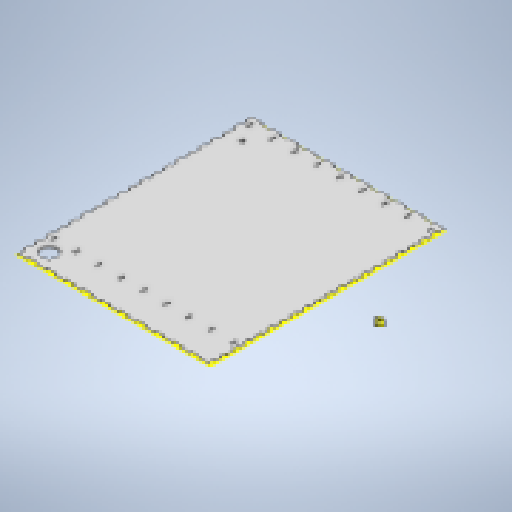
# Autodesk Inventor part: LedBoard
Saved by Autodesk Inventor 2024 (Build 280153000, 153)
## iProperties
Created: 2023-07-20
Part Number: LedBoard
Material: Generic
Document SubType Name: Modeling
Designer: Bruno
Density: 1 g/cm^3
Appearance: Default
Author: Bruno
Autodesk Inventor part; units mm, degrees
ref_plane "YZ Plane" through (0, 0, 0) normal (1, 0, 0) x (0, 1, 0)
ref_plane "XZ Plane" through (0, 0, 0) normal (0, 1, 0) x (-1, 0, 0)
ref_plane "XY Plane" through (0, 0, 0) normal (0, 0, 1) x (1, 0, 0)
sketch "Sketch1" plane through (0, 0, 0) normal (0, 1, 0) x (-1, 0, 0)
  line L0 (378.2704, -187.5) -> (378.2704, 177.5) projected
  line L1 (78.2704, -187.5) -> (378.2704, -187.5) projected
  line L2 (78.2704, 177.5) -> (78.2704, -187.5) projected
  line L3 (378.2704, 177.5) -> (78.2704, 177.5) projected
  line L4 (378.2704, 168.375) -> (378.2704, 177.5) projected
  line L5 (378.2704, 177.5) -> (375.2704, 177.5) projected
  line L6 (375.2704, 168.375) -> (375.2704, 177.5) projected
  line L7 (378.2704, 168.375) -> (375.2704, 168.375) projected
  line L8 (378.2704, 150.125) -> (378.2704, 159.25) projected
  line L9 (378.2704, 159.25) -> (375.2704, 159.25) projected
  line L10 (375.2704, 150.125) -> (375.2704, 159.25) projected
  line L11 (378.2704, 150.125) -> (375.2704, 150.125) projected
  line L12 (378.2704, 131.875) -> (378.2704, 141) projected
  line L13 (378.2704, 141) -> (375.2704, 141) projected
  line L14 (375.2704, 131.875) -> (375.2704, 141) projected
  line L15 (378.2704, 131.875) -> (375.2704, 131.875) projected
  line L16 (378.2704, 113.625) -> (378.2704, 122.75) projected
  line L17 (378.2704, 122.75) -> (375.2704, 122.75) projected
  line L18 (375.2704, 113.625) -> (375.2704, 122.75) projected
  line L19 (378.2704, 113.625) -> (375.2704, 113.625) projected
  line L20 (378.2704, 95.375) -> (378.2704, 104.5) projected
  line L21 (378.2704, 104.5) -> (375.2704, 104.5) projected
  line L22 (375.2704, 95.375) -> (375.2704, 104.5) projected
  line L23 (378.2704, 95.375) -> (375.2704, 95.375) projected
  line L24 (378.2704, 77.125) -> (378.2704, 86.25) projected
  line L25 (378.2704, 86.25) -> (375.2704, 86.25) projected
  line L26 (375.2704, 77.125) -> (375.2704, 86.25) projected
  line L27 (378.2704, 77.125) -> (375.2704, 77.125) projected
  line L28 (378.2704, 58.875) -> (378.2704, 68) projected
  line L29 (378.2704, 68) -> (375.2704, 68) projected
  line L30 (375.2704, 58.875) -> (375.2704, 68) projected
  line L31 (378.2704, 58.875) -> (375.2704, 58.875) projected
  line L32 (378.2704, 4.125) -> (378.2704, 13.25) projected
  line L33 (378.2704, 13.25) -> (375.2704, 13.25) projected
  line L34 (375.2704, 4.125) -> (375.2704, 13.25) projected
  line L35 (378.2704, 4.125) -> (375.2704, 4.125) projected
  line L36 (378.2704, 22.375) -> (378.2704, 31.5) projected
  line L37 (378.2704, 31.5) -> (375.2704, 31.5) projected
  line L38 (375.2704, 22.375) -> (375.2704, 31.5) projected
  line L39 (378.2704, 22.375) -> (375.2704, 22.375) projected
  line L40 (378.2704, 40.625) -> (378.2704, 49.75) projected
  line L41 (378.2704, 49.75) -> (375.2704, 49.75) projected
  line L42 (375.2704, 40.625) -> (375.2704, 49.75) projected
  line L43 (378.2704, 40.625) -> (375.2704, 40.625) projected
  line L44 (378.2704, -87.125) -> (378.2704, -78) projected
  line L45 (378.2704, -78) -> (375.2704, -78) projected
  line L46 (375.2704, -87.125) -> (375.2704, -78) projected
  line L47 (378.2704, -87.125) -> (375.2704, -87.125) projected
  line L48 (378.2704, -68.875) -> (378.2704, -59.75) projected
  line L49 (378.2704, -59.75) -> (375.2704, -59.75) projected
  line L50 (375.2704, -68.875) -> (375.2704, -59.75) projected
  line L51 (378.2704, -68.875) -> (375.2704, -68.875) projected
  line L52 (378.2704, -50.625) -> (378.2704, -41.5) projected
  line L53 (378.2704, -41.5) -> (375.2704, -41.5) projected
  line L54 (375.2704, -50.625) -> (375.2704, -41.5) projected
  line L55 (378.2704, -50.625) -> (375.2704, -50.625) projected
  line L56 (378.2704, -32.375) -> (378.2704, -23.25) projected
  line L57 (378.2704, -23.25) -> (375.2704, -23.25) projected
  line L58 (375.2704, -32.375) -> (375.2704, -23.25) projected
  line L59 (378.2704, -32.375) -> (375.2704, -32.375) projected
  line L60 (378.2704, -14.125) -> (378.2704, -5) projected
  line L61 (378.2704, -5) -> (375.2704, -5) projected
  line L62 (375.2704, -14.125) -> (375.2704, -5) projected
  line L63 (378.2704, -14.125) -> (375.2704, -14.125) projected
  line L64 (378.2704, -178.375) -> (378.2704, -169.25) projected
  line L65 (378.2704, -169.25) -> (375.2704, -169.25) projected
  line L66 (375.2704, -178.375) -> (375.2704, -169.25) projected
  line L67 (378.2704, -178.375) -> (375.2704, -178.375) projected
  line L68 (378.2704, -160.125) -> (378.2704, -151) projected
  line L69 (378.2704, -151) -> (375.2704, -151) projected
  line L70 (375.2704, -160.125) -> (375.2704, -151) projected
  line L71 (378.2704, -160.125) -> (375.2704, -160.125) projected
  line L72 (378.2704, -141.875) -> (378.2704, -132.75) projected
  line L73 (378.2704, -132.75) -> (375.2704, -132.75) projected
  line L74 (375.2704, -141.875) -> (375.2704, -132.75) projected
  line L75 (378.2704, -141.875) -> (375.2704, -141.875) projected
  line L76 (378.2704, -123.625) -> (378.2704, -114.5) projected
  line L77 (378.2704, -114.5) -> (375.2704, -114.5) projected
  line L78 (375.2704, -123.625) -> (375.2704, -114.5) projected
  line L79 (378.2704, -123.625) -> (375.2704, -123.625) projected
  line L80 (378.2704, -105.375) -> (378.2704, -96.25) projected
  line L81 (378.2704, -96.25) -> (375.2704, -96.25) projected
  line L82 (375.2704, -105.375) -> (375.2704, -96.25) projected
  line L83 (378.2704, -105.375) -> (375.2704, -105.375) projected
  line L84 (361.2704, -184.5) -> (347.2704, -184.5) projected
  line L85 (347.2704, -184.5) -> (347.2704, -187.5) projected
  line L86 (361.2704, -187.5) -> (347.2704, -187.5) projected
  line L87 (361.2704, -184.5) -> (361.2704, -187.5) projected
  line L88 (333.2704, -184.5) -> (319.2704, -184.5) projected
  line L89 (319.2704, -184.5) -> (319.2704, -187.5) projected
  line L90 (333.2704, -187.5) -> (319.2704, -187.5) projected
  line L91 (333.2704, -184.5) -> (333.2704, -187.5) projected
  line L92 (305.2704, -184.5) -> (291.2704, -184.5) projected
  line L93 (291.2704, -184.5) -> (291.2704, -187.5) projected
  line L94 (305.2704, -187.5) -> (291.2704, -187.5) projected
  line L95 (305.2704, -184.5) -> (305.2704, -187.5) projected
  line L96 (277.2704, -184.5) -> (263.2704, -184.5) projected
  line L97 (263.2704, -184.5) -> (263.2704, -187.5) projected
  line L98 (277.2704, -187.5) -> (263.2704, -187.5) projected
  line L99 (277.2704, -184.5) -> (277.2704, -187.5) projected
  line L100 (249.2704, -184.5) -> (235.2704, -184.5) projected
  line L101 (235.2704, -184.5) -> (235.2704, -187.5) projected
  line L102 (249.2704, -187.5) -> (235.2704, -187.5) projected
  line L103 (249.2704, -184.5) -> (249.2704, -187.5) projected
  line L104 (221.2704, -184.5) -> (207.2704, -184.5) projected
  line L105 (207.2704, -184.5) -> (207.2704, -187.5) projected
  line L106 (221.2704, -187.5) -> (207.2704, -187.5) projected
  line L107 (221.2704, -184.5) -> (221.2704, -187.5) projected
  line L108 (193.2704, -184.5) -> (179.2704, -184.5) projected
  line L109 (179.2704, -184.5) -> (179.2704, -187.5) projected
  line L110 (193.2704, -187.5) -> (179.2704, -187.5) projected
  line L111 (193.2704, -184.5) -> (193.2704, -187.5) projected
  line L112 (165.2704, -184.5) -> (151.2704, -184.5) projected
  line L113 (151.2704, -184.5) -> (151.2704, -187.5) projected
  line L114 (165.2704, -187.5) -> (151.2704, -187.5) projected
  line L115 (165.2704, -184.5) -> (165.2704, -187.5) projected
  line L116 (137.2704, -184.5) -> (123.2704, -184.5) projected
  line L117 (123.2704, -184.5) -> (123.2704, -187.5) projected
  line L118 (137.2704, -187.5) -> (123.2704, -187.5) projected
  line L119 (137.2704, -184.5) -> (137.2704, -187.5) projected
  line L120 (109.2704, -184.5) -> (95.2704, -184.5) projected
  line L121 (95.2704, -184.5) -> (95.2704, -187.5) projected
  line L122 (109.2704, -187.5) -> (95.2704, -187.5) projected
  line L123 (109.2704, -184.5) -> (109.2704, -187.5) projected
  line L124 (81.2704, -178.375) -> (81.2704, -169.25) projected
  line L125 (81.2704, -169.25) -> (78.2704, -169.25) projected
  line L126 (78.2704, -178.375) -> (78.2704, -169.25) projected
  line L127 (81.2704, -178.375) -> (78.2704, -178.375) projected
  line L128 (81.2704, -160.125) -> (81.2704, -151) projected
  line L129 (81.2704, -151) -> (78.2704, -151) projected
  line L130 (78.2704, -160.125) -> (78.2704, -151) projected
  line L131 (81.2704, -160.125) -> (78.2704, -160.125) projected
  line L132 (81.2704, -141.875) -> (81.2704, -132.75) projected
  line L133 (81.2704, -132.75) -> (78.2704, -132.75) projected
  line L134 (78.2704, -141.875) -> (78.2704, -132.75) projected
  line L135 (81.2704, -141.875) -> (78.2704, -141.875) projected
  line L136 (81.2704, -123.625) -> (81.2704, -114.5) projected
  line L137 (81.2704, -114.5) -> (78.2704, -114.5) projected
  line L138 (78.2704, -123.625) -> (78.2704, -114.5) projected
  line L139 (81.2704, -123.625) -> (78.2704, -123.625) projected
  line L140 (81.2704, -105.375) -> (81.2704, -96.25) projected
  line L141 (81.2704, -96.25) -> (78.2704, -96.25) projected
  line L142 (78.2704, -105.375) -> (78.2704, -96.25) projected
  line L143 (81.2704, -105.375) -> (78.2704, -105.375) projected
  line L144 (81.2704, -87.125) -> (81.2704, -78) projected
  line L145 (81.2704, -78) -> (78.2704, -78) projected
  line L146 (78.2704, -87.125) -> (78.2704, -78) projected
  line L147 (81.2704, -87.125) -> (78.2704, -87.125) projected
  line L148 (81.2704, -68.875) -> (81.2704, -59.75) projected
  line L149 (81.2704, -59.75) -> (78.2704, -59.75) projected
  line L150 (78.2704, -68.875) -> (78.2704, -59.75) projected
  line L151 (81.2704, -68.875) -> (78.2704, -68.875) projected
  line L152 (81.2704, -50.625) -> (81.2704, -41.5) projected
  line L153 (81.2704, -41.5) -> (78.2704, -41.5) projected
  line L154 (78.2704, -50.625) -> (78.2704, -41.5) projected
  line L155 (81.2704, -50.625) -> (78.2704, -50.625) projected
  line L156 (81.2704, -32.375) -> (81.2704, -23.25) projected
  line L157 (81.2704, -23.25) -> (78.2704, -23.25) projected
  line L158 (78.2704, -32.375) -> (78.2704, -23.25) projected
  line L159 (81.2704, -32.375) -> (78.2704, -32.375) projected
  line L160 (81.2704, -14.125) -> (81.2704, -5) projected
  line L161 (81.2704, -5) -> (78.2704, -5) projected
  line L162 (78.2704, -14.125) -> (78.2704, -5) projected
  line L163 (81.2704, -14.125) -> (78.2704, -14.125) projected
  line L164 (81.2704, 4.125) -> (81.2704, 13.25) projected
  line L165 (81.2704, 13.25) -> (78.2704, 13.25) projected
  line L166 (78.2704, 4.125) -> (78.2704, 13.25) projected
  line L167 (81.2704, 4.125) -> (78.2704, 4.125) projected
  line L168 (81.2704, 22.375) -> (81.2704, 31.5) projected
  line L169 (81.2704, 31.5) -> (78.2704, 31.5) projected
  line L170 (78.2704, 22.375) -> (78.2704, 31.5) projected
  line L171 (81.2704, 22.375) -> (78.2704, 22.375) projected
  line L172 (81.2704, 40.625) -> (81.2704, 49.75) projected
  line L173 (81.2704, 49.75) -> (78.2704, 49.75) projected
  line L174 (78.2704, 40.625) -> (78.2704, 49.75) projected
  line L175 (81.2704, 40.625) -> (78.2704, 40.625) projected
  line L176 (81.2704, 58.875) -> (81.2704, 68) projected
  line L177 (81.2704, 68) -> (78.2704, 68) projected
  line L178 (78.2704, 58.875) -> (78.2704, 68) projected
  line L179 (81.2704, 58.875) -> (78.2704, 58.875) projected
  line L180 (81.2704, 77.125) -> (81.2704, 86.25) projected
  line L181 (81.2704, 86.25) -> (78.2704, 86.25) projected
  line L182 (78.2704, 77.125) -> (78.2704, 86.25) projected
  line L183 (81.2704, 77.125) -> (78.2704, 77.125) projected
  line L184 (81.2704, 95.375) -> (81.2704, 104.5) projected
  line L185 (81.2704, 104.5) -> (78.2704, 104.5) projected
  line L186 (78.2704, 95.375) -> (78.2704, 104.5) projected
  line L187 (81.2704, 95.375) -> (78.2704, 95.375) projected
  line L188 (81.2704, 113.625) -> (81.2704, 122.75) projected
  line L189 (81.2704, 122.75) -> (78.2704, 122.75) projected
  line L190 (78.2704, 113.625) -> (78.2704, 122.75) projected
  line L191 (81.2704, 113.625) -> (78.2704, 113.625) projected
  line L192 (81.2704, 131.875) -> (81.2704, 141) projected
  line L193 (81.2704, 141) -> (78.2704, 141) projected
  line L194 (78.2704, 131.875) -> (78.2704, 141) projected
  line L195 (81.2704, 131.875) -> (78.2704, 131.875) projected
  line L196 (81.2704, 150.125) -> (81.2704, 159.25) projected
  line L197 (81.2704, 159.25) -> (78.2704, 159.25) projected
  line L198 (78.2704, 150.125) -> (78.2704, 159.25) projected
  line L199 (81.2704, 150.125) -> (78.2704, 150.125) projected
  line L200 (81.2704, 168.375) -> (81.2704, 177.5) projected
  line L201 (81.2704, 177.5) -> (78.2704, 177.5) projected
  line L202 (78.2704, 168.375) -> (78.2704, 177.5) projected
  line L203 (81.2704, 168.375) -> (78.2704, 168.375) projected
  line L204 (361.2704, 177.5) -> (347.2704, 177.5) projected
  line L205 (347.2704, 177.5) -> (347.2704, 174.5) projected
  line L206 (361.2704, 174.5) -> (347.2704, 174.5) projected
  line L207 (361.2704, 177.5) -> (361.2704, 174.5) projected
  line L208 (333.2704, 177.5) -> (319.2704, 177.5) projected
  line L209 (319.2704, 177.5) -> (319.2704, 174.5) projected
  line L210 (333.2704, 174.5) -> (319.2704, 174.5) projected
  line L211 (333.2704, 177.5) -> (333.2704, 174.5) projected
  line L212 (305.2704, 177.5) -> (291.2704, 177.5) projected
  line L213 (291.2704, 177.5) -> (291.2704, 174.5) projected
  line L214 (305.2704, 174.5) -> (291.2704, 174.5) projected
  line L215 (305.2704, 177.5) -> (305.2704, 174.5) projected
  line L216 (277.2704, 177.5) -> (263.2704, 177.5) projected
  line L217 (263.2704, 177.5) -> (263.2704, 174.5) projected
  line L218 (277.2704, 174.5) -> (263.2704, 174.5) projected
  line L219 (277.2704, 177.5) -> (277.2704, 174.5) projected
  line L220 (249.2704, 177.5) -> (235.2704, 177.5) projected
  line L221 (235.2704, 177.5) -> (235.2704, 174.5) projected
  line L222 (249.2704, 174.5) -> (235.2704, 174.5) projected
  line L223 (249.2704, 177.5) -> (249.2704, 174.5) projected
  line L224 (221.2704, 177.5) -> (207.2704, 177.5) projected
  line L225 (207.2704, 177.5) -> (207.2704, 174.5) projected
  line L226 (221.2704, 174.5) -> (207.2704, 174.5) projected
  line L227 (221.2704, 177.5) -> (221.2704, 174.5) projected
  line L228 (193.2704, 177.5) -> (179.2704, 177.5) projected
  line L229 (179.2704, 177.5) -> (179.2704, 174.5) projected
  line L230 (193.2704, 174.5) -> (179.2704, 174.5) projected
  line L231 (193.2704, 177.5) -> (193.2704, 174.5) projected
  line L232 (165.2704, 177.5) -> (151.2704, 177.5) projected
  line L233 (151.2704, 177.5) -> (151.2704, 174.5) projected
  line L234 (165.2704, 174.5) -> (151.2704, 174.5) projected
  line L235 (165.2704, 177.5) -> (165.2704, 174.5) projected
  line L236 (137.2704, 177.5) -> (123.2704, 177.5) projected
  line L237 (123.2704, 177.5) -> (123.2704, 174.5) projected
  line L238 (137.2704, 174.5) -> (123.2704, 174.5) projected
  line L239 (137.2704, 177.5) -> (137.2704, 174.5) projected
  line L240 (109.2704, 177.5) -> (95.2704, 177.5) projected
  line L241 (95.2704, 177.5) -> (95.2704, 174.5) projected
  line L242 (109.2704, 174.5) -> (95.2704, 174.5) projected
  line L243 (109.2704, 177.5) -> (109.2704, 174.5) projected
  constraints: 4 other
extrude "Extrusion1" add sketch "Sketch1" along normal blind 3 contours L1 L87 L84 L85 L91 L88 L89 L95 L92 L93 L99 L96 L97 L103 L100 L101 L107 L104 L105 L111 L108 L109 L115 L112 L113 L119 L116 L117 L123 L120 L121 L2 L127 L124 L125 L131 L128 L129 L135 L132 L133 L139 L136 L137 L143 L140 L141 L147 L144 L145 L151 L148 L149 L155 L152 L153 L159 L156 L157 L163 L160 L161 L167 L164 L165 L171 L168 L169 L175 L172 L173 L179 L176 L177 L183 L180 L181 L187 L184 L185 L191 L188 L189 L195 L192 L193 L199 L196 L197 L203 L200 L3 L241 L242 L243 L237 L238 L239 L233 L234 L235 L229 L230 L231 L225 L226 L227 L221 L222 L223 L217 L218 L219 L213 L214 L215 L209 L210 L211 L205 L206 L207 L6 L7 L0 L9 L10 L11 L13 L14 L15 L17 L18 L19 L21 L22 L23 L25 L26 L27 L29 L30 L31 L41 L42 L43 L37 L38 L39 L33 L34 L35 L61 L62 L63 L57 L58 L59 L53 L54 L55 L49 L50 L51 L45 L46 L47 L81 L82 L83 L77 L78 L79 L73 L74 L75 L69 L70 L71 L65 L66 L67
sketch "Sketch3" plane through (0, 0, 0) normal (0, -1, 0) x (1, 0, 0)
  line L0 (-369.7704, 134.05) -> (-369.7704, 126.05) projected
  line L1 (-369.7704, 126.05) -> (-366.7704, 126.05) projected
  line L2 (-366.7704, 134.05) -> (-366.7704, 126.05) projected
  line L3 (-369.7704, 134.05) -> (-366.7704, 134.05) projected
  line L4 (-334.7704, 134.05) -> (-334.7704, 126.05) projected
  line L5 (-334.7704, 126.05) -> (-331.7704, 126.05) projected
  line L6 (-331.7704, 134.05) -> (-331.7704, 126.05) projected
  line L7 (-334.7704, 134.05) -> (-331.7704, 134.05) projected
  line L8 (-299.7704, 134.05) -> (-299.7704, 126.05) projected
  line L9 (-299.7704, 126.05) -> (-296.7704, 126.05) projected
  line L10 (-296.7704, 134.05) -> (-296.7704, 126.05) projected
  line L11 (-299.7704, 134.05) -> (-296.7704, 134.05) projected
  line L12 (-264.7704, 134.05) -> (-264.7704, 126.05) projected
  line L13 (-264.7704, 126.05) -> (-261.7704, 126.05) projected
  line L14 (-261.7704, 134.05) -> (-261.7704, 126.05) projected
  line L15 (-264.7704, 134.05) -> (-261.7704, 134.05) projected
  line L16 (-229.7704, 134.05) -> (-229.7704, 126.05) projected
  line L17 (-229.7704, 126.05) -> (-226.7704, 126.05) projected
  line L18 (-226.7704, 134.05) -> (-226.7704, 126.05) projected
  line L19 (-229.7704, 134.05) -> (-226.7704, 134.05) projected
  line L20 (-194.7704, 134.05) -> (-194.7704, 126.05) projected
  line L21 (-194.7704, 126.05) -> (-191.7704, 126.05) projected
  line L22 (-191.7704, 134.05) -> (-191.7704, 126.05) projected
  line L23 (-194.7704, 134.05) -> (-191.7704, 134.05) projected
  line L24 (-159.7704, 134.05) -> (-159.7704, 126.05) projected
  line L25 (-159.7704, 126.05) -> (-156.7704, 126.05) projected
  line L26 (-156.7704, 134.05) -> (-156.7704, 126.05) projected
  line L27 (-159.7704, 134.05) -> (-156.7704, 134.05) projected
  line L28 (-124.7704, 134.05) -> (-124.7704, 126.05) projected
  line L29 (-124.7704, 126.05) -> (-121.7704, 126.05) projected
  line L30 (-121.7704, 134.05) -> (-121.7704, 126.05) projected
  line L31 (-124.7704, 134.05) -> (-121.7704, 134.05) projected
  line L32 (-89.7704, 134.05) -> (-89.7704, 126.05) projected
  line L33 (-89.7704, 126.05) -> (-86.7704, 126.05) projected
  line L34 (-86.7704, 134.05) -> (-86.7704, 126.05) projected
  line L35 (-89.7704, 134.05) -> (-86.7704, 134.05) projected
  line L36 (-369.7704, -171.05) -> (-369.7704, -179.05) projected
  line L37 (-369.7704, -179.05) -> (-366.7704, -179.05) projected
  line L38 (-366.7704, -171.05) -> (-366.7704, -179.05) projected
  line L39 (-369.7704, -171.05) -> (-366.7704, -171.05) projected
  line L40 (-334.7704, -171.05) -> (-334.7704, -179.05) projected
  line L41 (-334.7704, -179.05) -> (-331.7704, -179.05) projected
  line L42 (-331.7704, -171.05) -> (-331.7704, -179.05) projected
  line L43 (-334.7704, -171.05) -> (-331.7704, -171.05) projected
  line L44 (-299.7704, -171.05) -> (-299.7704, -179.05) projected
  line L45 (-299.7704, -179.05) -> (-296.7704, -179.05) projected
  line L46 (-296.7704, -171.05) -> (-296.7704, -179.05) projected
  line L47 (-299.7704, -171.05) -> (-296.7704, -171.05) projected
  line L48 (-264.7704, -171.05) -> (-264.7704, -179.05) projected
  line L49 (-264.7704, -179.05) -> (-261.7704, -179.05) projected
  line L50 (-261.7704, -171.05) -> (-261.7704, -179.05) projected
  line L51 (-264.7704, -171.05) -> (-261.7704, -171.05) projected
  line L52 (-229.7704, -171.05) -> (-229.7704, -179.05) projected
  line L53 (-229.7704, -179.05) -> (-226.7704, -179.05) projected
  line L54 (-226.7704, -171.05) -> (-226.7704, -179.05) projected
  line L55 (-229.7704, -171.05) -> (-226.7704, -171.05) projected
  line L56 (-194.7704, -171.05) -> (-194.7704, -179.05) projected
  line L57 (-194.7704, -179.05) -> (-191.7704, -179.05) projected
  line L58 (-191.7704, -171.05) -> (-191.7704, -179.05) projected
  line L59 (-194.7704, -171.05) -> (-191.7704, -171.05) projected
  line L60 (-159.7704, -171.05) -> (-159.7704, -179.05) projected
  line L61 (-159.7704, -179.05) -> (-156.7704, -179.05) projected
  line L62 (-156.7704, -171.05) -> (-156.7704, -179.05) projected
  line L63 (-159.7704, -171.05) -> (-156.7704, -171.05) projected
  line L64 (-124.7704, -171.05) -> (-124.7704, -179.05) projected
  line L65 (-124.7704, -179.05) -> (-121.7704, -179.05) projected
  line L66 (-121.7704, -171.05) -> (-121.7704, -179.05) projected
  line L67 (-124.7704, -171.05) -> (-121.7704, -171.05) projected
  line L68 (-89.7704, -171.05) -> (-89.7704, -179.05) projected
  line L69 (-89.7704, -179.05) -> (-86.7704, -179.05) projected
  line L70 (-86.7704, -171.05) -> (-86.7704, -179.05) projected
  line L71 (-89.7704, -171.05) -> (-86.7704, -171.05) projected
  point P0 (0, 0)
extrude "Extrusion3" cut sketch "Sketch3" against normal up to surface (3 mm away)
sketch "Sketch4" plane through (0, 3, 0) normal (0, 1, 0) x (1, 0, 0)
  line L0 (-353.2704, -152.5) -> (-378.2704, -152.5) construction
  line L1 (-378.2704, -141) -> (-378.2704, -150.125) projected
  line L2 (-353.2704, -152.5) -> (-353.2704, -177.5) construction
  line L3 (-375.2704, -177.5) -> (-361.2704, -177.5) projected
  circle A0 centre (-229.7704, -152.5) radius 12.5
  line L4 (-353.2704, -152.5) -> (-229.7704, -152.5) construction
  line L5 (-229.7704, -152.5) -> (-106.2704, -152.5) construction
  line L6 (-106.2704, -152.5) -> (-81.2704, -152.5) construction
  line L7 (-81.2704, -159.25) -> (-81.2704, -150.125) projected
  point P0 (0, 0)
  point P1 (-78.2704, -177.5)
  dimension "d17" = 25
  dimension "d18" = 25
  dimension "d32" = 25
  constraints: 10 end point, 3 collinear, 3 point on line, 2 horizontal, 2 perpendicular, 1 centre point
  measures "d17" distance of L0.start L2.end
  measures "d18" distance of L0.start L0.end
  measures "d32" diameter of A0
extrude "Extrusion4" cut sketch "Sketch4" against normal through all
sketch "Sketch5" plane through (0, 3, 0) normal (0, 1, 0) x (1, 0, 0)
  line L0 (-353.5204, 147.75) -> (-348.0204, 147.75)
  line L1 (-348.0204, 147.75) -> (-348.0204, 142.25)
  line L2 (-348.0204, 142.25) -> (-353.5204, 142.25)
  line L3 (-353.5204, 142.25) -> (-353.5204, 147.75)
  line L4 (-353.5204, 145) -> (-348.0204, 145) construction
  line L5 (-350.7704, 142.25) -> (-350.7704, 147.75) construction
  line L6 (-366.7704, 142.5) -> (-366.7704, 147.5) projected
  line L7 (-353.2704, 161) -> (-348.2704, 161) projected
  line L8 (-318.5204, 147.75) -> (-313.0204, 147.75)
  line L9 (-313.0204, 147.75) -> (-313.0204, 142.25)
  line L10 (-313.0204, 142.25) -> (-318.5204, 142.25)
  line L11 (-318.5204, 142.25) -> (-318.5204, 147.75)
  line L12 (-318.5204, 145) -> (-313.0204, 145) construction
  line L13 (-315.7704, 142.25) -> (-315.7704, 147.75) construction
  line L14 (-283.5204, 147.75) -> (-278.0204, 147.75)
  line L15 (-278.0204, 147.75) -> (-278.0204, 142.25)
  line L16 (-278.0204, 142.25) -> (-283.5204, 142.25)
  line L17 (-283.5204, 142.25) -> (-283.5204, 147.75)
  line L18 (-283.5204, 145) -> (-278.0204, 145) construction
  line L19 (-280.7704, 142.25) -> (-280.7704, 147.75) construction
  line L20 (-248.5204, 147.75) -> (-243.0204, 147.75)
  line L21 (-243.0204, 147.75) -> (-243.0204, 142.25)
  line L22 (-243.0204, 142.25) -> (-248.5204, 142.25)
  line L23 (-248.5204, 142.25) -> (-248.5204, 147.75)
  line L24 (-248.5204, 145) -> (-243.0204, 145) construction
  line L25 (-245.7704, 142.25) -> (-245.7704, 147.75) construction
  line L26 (-213.5204, 147.75) -> (-208.0204, 147.75)
  line L27 (-208.0204, 147.75) -> (-208.0204, 142.25)
  line L28 (-208.0204, 142.25) -> (-213.5204, 142.25)
  line L29 (-213.5204, 142.25) -> (-213.5204, 147.75)
  line L30 (-213.5204, 145) -> (-208.0204, 145) construction
  line L31 (-210.7704, 142.25) -> (-210.7704, 147.75) construction
  line L32 (-178.5204, 147.75) -> (-173.0204, 147.75)
  line L33 (-173.0204, 147.75) -> (-173.0204, 142.25)
  line L34 (-173.0204, 142.25) -> (-178.5204, 142.25)
  line L35 (-178.5204, 142.25) -> (-178.5204, 147.75)
  line L36 (-178.5204, 145) -> (-173.0204, 145) construction
  line L37 (-175.7704, 142.25) -> (-175.7704, 147.75) construction
  line L38 (-143.5204, 147.75) -> (-138.0204, 147.75)
  line L39 (-138.0204, 147.75) -> (-138.0204, 142.25)
  line L40 (-138.0204, 142.25) -> (-143.5204, 142.25)
  line L41 (-143.5204, 142.25) -> (-143.5204, 147.75)
  line L42 (-143.5204, 145) -> (-138.0204, 145) construction
  line L43 (-140.7704, 142.25) -> (-140.7704, 147.75) construction
  line L44 (-108.5204, 147.75) -> (-103.0204, 147.75)
  line L45 (-103.0204, 147.75) -> (-103.0204, 142.25)
  line L46 (-103.0204, 142.25) -> (-108.5204, 142.25)
  line L47 (-108.5204, 142.25) -> (-108.5204, 147.75)
  line L48 (-108.5204, 145) -> (-103.0204, 145) construction
  line L49 (-105.7704, 142.25) -> (-105.7704, 147.75) construction
  line L50 (-353.5204, 112.75) -> (-348.0204, 112.75)
  line L51 (-348.0204, 112.75) -> (-348.0204, 107.25)
  line L52 (-348.0204, 107.25) -> (-353.5204, 107.25)
  line L53 (-353.5204, 107.25) -> (-353.5204, 112.75)
  line L54 (-353.5204, 110) -> (-348.0204, 110) construction
  line L55 (-350.7704, 107.25) -> (-350.7704, 112.75) construction
  line L56 (-318.5204, 112.75) -> (-313.0204, 112.75)
  line L57 (-313.0204, 112.75) -> (-313.0204, 107.25)
  line L58 (-313.0204, 107.25) -> (-318.5204, 107.25)
  line L59 (-318.5204, 107.25) -> (-318.5204, 112.75)
  line L60 (-318.5204, 110) -> (-313.0204, 110) construction
  line L61 (-315.7704, 107.25) -> (-315.7704, 112.75) construction
  line L62 (-283.5204, 112.75) -> (-278.0204, 112.75)
  line L63 (-278.0204, 112.75) -> (-278.0204, 107.25)
  line L64 (-278.0204, 107.25) -> (-283.5204, 107.25)
  line L65 (-283.5204, 107.25) -> (-283.5204, 112.75)
  line L66 (-283.5204, 110) -> (-278.0204, 110) construction
  line L67 (-280.7704, 107.25) -> (-280.7704, 112.75) construction
  line L68 (-248.5204, 112.75) -> (-243.0204, 112.75)
  line L69 (-243.0204, 112.75) -> (-243.0204, 107.25)
  line L70 (-243.0204, 107.25) -> (-248.5204, 107.25)
  line L71 (-248.5204, 107.25) -> (-248.5204, 112.75)
  line L72 (-248.5204, 110) -> (-243.0204, 110) construction
  line L73 (-245.7704, 107.25) -> (-245.7704, 112.75) construction
  line L74 (-213.5204, 112.75) -> (-208.0204, 112.75)
  line L75 (-208.0204, 112.75) -> (-208.0204, 107.25)
  line L76 (-208.0204, 107.25) -> (-213.5204, 107.25)
  line L77 (-213.5204, 107.25) -> (-213.5204, 112.75)
  line L78 (-213.5204, 110) -> (-208.0204, 110) construction
  line L79 (-210.7704, 107.25) -> (-210.7704, 112.75) construction
  line L80 (-178.5204, 112.75) -> (-173.0204, 112.75)
  line L81 (-173.0204, 112.75) -> (-173.0204, 107.25)
  line L82 (-173.0204, 107.25) -> (-178.5204, 107.25)
  line L83 (-178.5204, 107.25) -> (-178.5204, 112.75)
  line L84 (-178.5204, 110) -> (-173.0204, 110) construction
  line L85 (-175.7704, 107.25) -> (-175.7704, 112.75) construction
  line L86 (-143.5204, 112.75) -> (-138.0204, 112.75)
  line L87 (-138.0204, 112.75) -> (-138.0204, 107.25)
  line L88 (-138.0204, 107.25) -> (-143.5204, 107.25)
  line L89 (-143.5204, 107.25) -> (-143.5204, 112.75)
  line L90 (-143.5204, 110) -> (-138.0204, 110) construction
  line L91 (-140.7704, 107.25) -> (-140.7704, 112.75) construction
  line L92 (-108.5204, 112.75) -> (-103.0204, 112.75)
  line L93 (-103.0204, 112.75) -> (-103.0204, 107.25)
  line L94 (-103.0204, 107.25) -> (-108.5204, 107.25)
  line L95 (-108.5204, 107.25) -> (-108.5204, 112.75)
  line L96 (-108.5204, 110) -> (-103.0204, 110) construction
  line L97 (-105.7704, 107.25) -> (-105.7704, 112.75) construction
  line L98 (-353.5204, 77.75) -> (-348.0204, 77.75)
  line L99 (-348.0204, 77.75) -> (-348.0204, 72.25)
  line L100 (-348.0204, 72.25) -> (-353.5204, 72.25)
  line L101 (-353.5204, 72.25) -> (-353.5204, 77.75)
  line L102 (-353.5204, 75) -> (-348.0204, 75) construction
  line L103 (-350.7704, 72.25) -> (-350.7704, 77.75) construction
  line L104 (-318.5204, 77.75) -> (-313.0204, 77.75)
  line L105 (-313.0204, 77.75) -> (-313.0204, 72.25)
  line L106 (-313.0204, 72.25) -> (-318.5204, 72.25)
  line L107 (-318.5204, 72.25) -> (-318.5204, 77.75)
  line L108 (-318.5204, 75) -> (-313.0204, 75) construction
  line L109 (-315.7704, 72.25) -> (-315.7704, 77.75) construction
  line L110 (-283.5204, 77.75) -> (-278.0204, 77.75)
  line L111 (-278.0204, 77.75) -> (-278.0204, 72.25)
  line L112 (-278.0204, 72.25) -> (-283.5204, 72.25)
  line L113 (-283.5204, 72.25) -> (-283.5204, 77.75)
  line L114 (-283.5204, 75) -> (-278.0204, 75) construction
  line L115 (-280.7704, 72.25) -> (-280.7704, 77.75) construction
  line L116 (-248.5204, 77.75) -> (-243.0204, 77.75)
  line L117 (-243.0204, 77.75) -> (-243.0204, 72.25)
  line L118 (-243.0204, 72.25) -> (-248.5204, 72.25)
  line L119 (-248.5204, 72.25) -> (-248.5204, 77.75)
  line L120 (-248.5204, 75) -> (-243.0204, 75) construction
  line L121 (-245.7704, 72.25) -> (-245.7704, 77.75) construction
  line L122 (-213.5204, 77.75) -> (-208.0204, 77.75)
  line L123 (-208.0204, 77.75) -> (-208.0204, 72.25)
  line L124 (-208.0204, 72.25) -> (-213.5204, 72.25)
  line L125 (-213.5204, 72.25) -> (-213.5204, 77.75)
  line L126 (-213.5204, 75) -> (-208.0204, 75) construction
  line L127 (-210.7704, 72.25) -> (-210.7704, 77.75) construction
  line L128 (-178.5204, 77.75) -> (-173.0204, 77.75)
  line L129 (-173.0204, 77.75) -> (-173.0204, 72.25)
  line L130 (-173.0204, 72.25) -> (-178.5204, 72.25)
  line L131 (-178.5204, 72.25) -> (-178.5204, 77.75)
  line L132 (-178.5204, 75) -> (-173.0204, 75) construction
  line L133 (-175.7704, 72.25) -> (-175.7704, 77.75) construction
  line L134 (-143.5204, 77.75) -> (-138.0204, 77.75)
  line L135 (-138.0204, 77.75) -> (-138.0204, 72.25)
  line L136 (-138.0204, 72.25) -> (-143.5204, 72.25)
  line L137 (-143.5204, 72.25) -> (-143.5204, 77.75)
  line L138 (-143.5204, 75) -> (-138.0204, 75) construction
  line L139 (-140.7704, 72.25) -> (-140.7704, 77.75) construction
  line L140 (-108.5204, 77.75) -> (-103.0204, 77.75)
  line L141 (-103.0204, 77.75) -> (-103.0204, 72.25)
  line L142 (-103.0204, 72.25) -> (-108.5204, 72.25)
  line L143 (-108.5204, 72.25) -> (-108.5204, 77.75)
  line L144 (-108.5204, 75) -> (-103.0204, 75) construction
  line L145 (-105.7704, 72.25) -> (-105.7704, 77.75) construction
  line L146 (-353.5204, 42.75) -> (-348.0204, 42.75)
  line L147 (-348.0204, 42.75) -> (-348.0204, 37.25)
  line L148 (-348.0204, 37.25) -> (-353.5204, 37.25)
  line L149 (-353.5204, 37.25) -> (-353.5204, 42.75)
  line L150 (-353.5204, 40) -> (-348.0204, 40) construction
  line L151 (-350.7704, 37.25) -> (-350.7704, 42.75) construction
  line L152 (-318.5204, 42.75) -> (-313.0204, 42.75)
  line L153 (-313.0204, 42.75) -> (-313.0204, 37.25)
  line L154 (-313.0204, 37.25) -> (-318.5204, 37.25)
  line L155 (-318.5204, 37.25) -> (-318.5204, 42.75)
  line L156 (-318.5204, 40) -> (-313.0204, 40) construction
  line L157 (-315.7704, 37.25) -> (-315.7704, 42.75) construction
  line L158 (-283.5204, 42.75) -> (-278.0204, 42.75)
  line L159 (-278.0204, 42.75) -> (-278.0204, 37.25)
  line L160 (-278.0204, 37.25) -> (-283.5204, 37.25)
  line L161 (-283.5204, 37.25) -> (-283.5204, 42.75)
  line L162 (-283.5204, 40) -> (-278.0204, 40) construction
  line L163 (-280.7704, 37.25) -> (-280.7704, 42.75) construction
  line L164 (-248.5204, 42.75) -> (-243.0204, 42.75)
  line L165 (-243.0204, 42.75) -> (-243.0204, 37.25)
  line L166 (-243.0204, 37.25) -> (-248.5204, 37.25)
  line L167 (-248.5204, 37.25) -> (-248.5204, 42.75)
  line L168 (-248.5204, 40) -> (-243.0204, 40) construction
  line L169 (-245.7704, 37.25) -> (-245.7704, 42.75) construction
  line L170 (-213.5204, 42.75) -> (-208.0204, 42.75)
  line L171 (-208.0204, 42.75) -> (-208.0204, 37.25)
  line L172 (-208.0204, 37.25) -> (-213.5204, 37.25)
  line L173 (-213.5204, 37.25) -> (-213.5204, 42.75)
  line L174 (-213.5204, 40) -> (-208.0204, 40) construction
  line L175 (-210.7704, 37.25) -> (-210.7704, 42.75) construction
  line L176 (-178.5204, 42.75) -> (-173.0204, 42.75)
  line L177 (-173.0204, 42.75) -> (-173.0204, 37.25)
  line L178 (-173.0204, 37.25) -> (-178.5204, 37.25)
  line L179 (-178.5204, 37.25) -> (-178.5204, 42.75)
  line L180 (-178.5204, 40) -> (-173.0204, 40) construction
  line L181 (-175.7704, 37.25) -> (-175.7704, 42.75) construction
  line L182 (-143.5204, 42.75) -> (-138.0204, 42.75)
  line L183 (-138.0204, 42.75) -> (-138.0204, 37.25)
  line L184 (-138.0204, 37.25) -> (-143.5204, 37.25)
  line L185 (-143.5204, 37.25) -> (-143.5204, 42.75)
  line L186 (-143.5204, 40) -> (-138.0204, 40) construction
  line L187 (-140.7704, 37.25) -> (-140.7704, 42.75) construction
  line L188 (-108.5204, 42.75) -> (-103.0204, 42.75)
  line L189 (-103.0204, 42.75) -> (-103.0204, 37.25)
  line L190 (-103.0204, 37.25) -> (-108.5204, 37.25)
  line L191 (-108.5204, 37.25) -> (-108.5204, 42.75)
  line L192 (-108.5204, 40) -> (-103.0204, 40) construction
  line L193 (-105.7704, 37.25) -> (-105.7704, 42.75) construction
  line L194 (-353.5204, 7.75) -> (-348.0204, 7.75)
  line L195 (-348.0204, 7.75) -> (-348.0204, 2.25)
  line L196 (-348.0204, 2.25) -> (-353.5204, 2.25)
  line L197 (-353.5204, 2.25) -> (-353.5204, 7.75)
  line L198 (-353.5204, 5) -> (-348.0204, 5) construction
  line L199 (-350.7704, 2.25) -> (-350.7704, 7.75) construction
  line L200 (-318.5204, 7.75) -> (-313.0204, 7.75)
  line L201 (-313.0204, 7.75) -> (-313.0204, 2.25)
  line L202 (-313.0204, 2.25) -> (-318.5204, 2.25)
  line L203 (-318.5204, 2.25) -> (-318.5204, 7.75)
  line L204 (-318.5204, 5) -> (-313.0204, 5) construction
  line L205 (-315.7704, 2.25) -> (-315.7704, 7.75) construction
  line L206 (-283.5204, 7.75) -> (-278.0204, 7.75)
  line L207 (-278.0204, 7.75) -> (-278.0204, 2.25)
  line L208 (-278.0204, 2.25) -> (-283.5204, 2.25)
  line L209 (-283.5204, 2.25) -> (-283.5204, 7.75)
  line L210 (-283.5204, 5) -> (-278.0204, 5) construction
  line L211 (-280.7704, 2.25) -> (-280.7704, 7.75) construction
  line L212 (-248.5204, 7.75) -> (-243.0204, 7.75)
  line L213 (-243.0204, 7.75) -> (-243.0204, 2.25)
  line L214 (-243.0204, 2.25) -> (-248.5204, 2.25)
  line L215 (-248.5204, 2.25) -> (-248.5204, 7.75)
  line L216 (-248.5204, 5) -> (-243.0204, 5) construction
  line L217 (-245.7704, 2.25) -> (-245.7704, 7.75) construction
  line L218 (-213.5204, 7.75) -> (-208.0204, 7.75)
  line L219 (-208.0204, 7.75) -> (-208.0204, 2.25)
  line L220 (-208.0204, 2.25) -> (-213.5204, 2.25)
  line L221 (-213.5204, 2.25) -> (-213.5204, 7.75)
  line L222 (-213.5204, 5) -> (-208.0204, 5) construction
  line L223 (-210.7704, 2.25) -> (-210.7704, 7.75) construction
  line L224 (-178.5204, 7.75) -> (-173.0204, 7.75)
  line L225 (-173.0204, 7.75) -> (-173.0204, 2.25)
  line L226 (-173.0204, 2.25) -> (-178.5204, 2.25)
  line L227 (-178.5204, 2.25) -> (-178.5204, 7.75)
  line L228 (-178.5204, 5) -> (-173.0204, 5) construction
  line L229 (-175.7704, 2.25) -> (-175.7704, 7.75) construction
  line L230 (-143.5204, 7.75) -> (-138.0204, 7.75)
  line L231 (-138.0204, 7.75) -> (-138.0204, 2.25)
  line L232 (-138.0204, 2.25) -> (-143.5204, 2.25)
  line L233 (-143.5204, 2.25) -> (-143.5204, 7.75)
  line L234 (-143.5204, 5) -> (-138.0204, 5) construction
  line L235 (-140.7704, 2.25) -> (-140.7704, 7.75) construction
  line L236 (-108.5204, 7.75) -> (-103.0204, 7.75)
  line L237 (-103.0204, 7.75) -> (-103.0204, 2.25)
  line L238 (-103.0204, 2.25) -> (-108.5204, 2.25)
  line L239 (-108.5204, 2.25) -> (-108.5204, 7.75)
  line L240 (-108.5204, 5) -> (-103.0204, 5) construction
  line L241 (-105.7704, 2.25) -> (-105.7704, 7.75) construction
  line L242 (-353.5204, -27.25) -> (-348.0204, -27.25)
  line L243 (-348.0204, -27.25) -> (-348.0204, -32.75)
  line L244 (-348.0204, -32.75) -> (-353.5204, -32.75)
  line L245 (-353.5204, -32.75) -> (-353.5204, -27.25)
  line L246 (-353.5204, -30) -> (-348.0204, -30) construction
  line L247 (-350.7704, -32.75) -> (-350.7704, -27.25) construction
  line L248 (-318.5204, -27.25) -> (-313.0204, -27.25)
  line L249 (-313.0204, -27.25) -> (-313.0204, -32.75)
  line L250 (-313.0204, -32.75) -> (-318.5204, -32.75)
  line L251 (-318.5204, -32.75) -> (-318.5204, -27.25)
  line L252 (-318.5204, -30) -> (-313.0204, -30) construction
  line L253 (-315.7704, -32.75) -> (-315.7704, -27.25) construction
  line L254 (-283.5204, -27.25) -> (-278.0204, -27.25)
  line L255 (-278.0204, -27.25) -> (-278.0204, -32.75)
  line L256 (-278.0204, -32.75) -> (-283.5204, -32.75)
  line L257 (-283.5204, -32.75) -> (-283.5204, -27.25)
  line L258 (-283.5204, -30) -> (-278.0204, -30) construction
  line L259 (-280.7704, -32.75) -> (-280.7704, -27.25) construction
  line L260 (-248.5204, -27.25) -> (-243.0204, -27.25)
  line L261 (-243.0204, -27.25) -> (-243.0204, -32.75)
  line L262 (-243.0204, -32.75) -> (-248.5204, -32.75)
  line L263 (-248.5204, -32.75) -> (-248.5204, -27.25)
  line L264 (-248.5204, -30) -> (-243.0204, -30) construction
  line L265 (-245.7704, -32.75) -> (-245.7704, -27.25) construction
  line L266 (-213.5204, -27.25) -> (-208.0204, -27.25)
  line L267 (-208.0204, -27.25) -> (-208.0204, -32.75)
  line L268 (-208.0204, -32.75) -> (-213.5204, -32.75)
  line L269 (-213.5204, -32.75) -> (-213.5204, -27.25)
  line L270 (-213.5204, -30) -> (-208.0204, -30) construction
  line L271 (-210.7704, -32.75) -> (-210.7704, -27.25) construction
  line L272 (-178.5204, -27.25) -> (-173.0204, -27.25)
  line L273 (-173.0204, -27.25) -> (-173.0204, -32.75)
  line L274 (-173.0204, -32.75) -> (-178.5204, -32.75)
  line L275 (-178.5204, -32.75) -> (-178.5204, -27.25)
  line L276 (-178.5204, -30) -> (-173.0204, -30) construction
  line L277 (-175.7704, -32.75) -> (-175.7704, -27.25) construction
  line L278 (-143.5204, -27.25) -> (-138.0204, -27.25)
  line L279 (-138.0204, -27.25) -> (-138.0204, -32.75)
  line L280 (-138.0204, -32.75) -> (-143.5204, -32.75)
  line L281 (-143.5204, -32.75) -> (-143.5204, -27.25)
  line L282 (-143.5204, -30) -> (-138.0204, -30) construction
  line L283 (-140.7704, -32.75) -> (-140.7704, -27.25) construction
  line L284 (-108.5204, -27.25) -> (-103.0204, -27.25)
  line L285 (-103.0204, -27.25) -> (-103.0204, -32.75)
  line L286 (-103.0204, -32.75) -> (-108.5204, -32.75)
  line L287 (-108.5204, -32.75) -> (-108.5204, -27.25)
  line L288 (-108.5204, -30) -> (-103.0204, -30) construction
  line L289 (-105.7704, -32.75) -> (-105.7704, -27.25) construction
  line L290 (-353.5204, -62.25) -> (-348.0204, -62.25)
  line L291 (-348.0204, -62.25) -> (-348.0204, -67.75)
  line L292 (-348.0204, -67.75) -> (-353.5204, -67.75)
  line L293 (-353.5204, -67.75) -> (-353.5204, -62.25)
  line L294 (-353.5204, -65) -> (-348.0204, -65) construction
  line L295 (-350.7704, -67.75) -> (-350.7704, -62.25) construction
  line L296 (-318.5204, -62.25) -> (-313.0204, -62.25)
  line L297 (-313.0204, -62.25) -> (-313.0204, -67.75)
  line L298 (-313.0204, -67.75) -> (-318.5204, -67.75)
  line L299 (-318.5204, -67.75) -> (-318.5204, -62.25)
  line L300 (-318.5204, -65) -> (-313.0204, -65) construction
  line L301 (-315.7704, -67.75) -> (-315.7704, -62.25) construction
  line L302 (-283.5204, -62.25) -> (-278.0204, -62.25)
  line L303 (-278.0204, -62.25) -> (-278.0204, -67.75)
  line L304 (-278.0204, -67.75) -> (-283.5204, -67.75)
  line L305 (-283.5204, -67.75) -> (-283.5204, -62.25)
  line L306 (-283.5204, -65) -> (-278.0204, -65) construction
  line L307 (-280.7704, -67.75) -> (-280.7704, -62.25) construction
  line L308 (-248.5204, -62.25) -> (-243.0204, -62.25)
  line L309 (-243.0204, -62.25) -> (-243.0204, -67.75)
  line L310 (-243.0204, -67.75) -> (-248.5204, -67.75)
  line L311 (-248.5204, -67.75) -> (-248.5204, -62.25)
  line L312 (-248.5204, -65) -> (-243.0204, -65) construction
  line L313 (-245.7704, -67.75) -> (-245.7704, -62.25) construction
  line L314 (-213.5204, -62.25) -> (-208.0204, -62.25)
  line L315 (-208.0204, -62.25) -> (-208.0204, -67.75)
  line L316 (-208.0204, -67.75) -> (-213.5204, -67.75)
  line L317 (-213.5204, -67.75) -> (-213.5204, -62.25)
  line L318 (-213.5204, -65) -> (-208.0204, -65) construction
  line L319 (-210.7704, -67.75) -> (-210.7704, -62.25) construction
  line L320 (-178.5204, -62.25) -> (-173.0204, -62.25)
  line L321 (-173.0204, -62.25) -> (-173.0204, -67.75)
  line L322 (-173.0204, -67.75) -> (-178.5204, -67.75)
  line L323 (-178.5204, -67.75) -> (-178.5204, -62.25)
  line L324 (-178.5204, -65) -> (-173.0204, -65) construction
  line L325 (-175.7704, -67.75) -> (-175.7704, -62.25) construction
  line L326 (-143.5204, -62.25) -> (-138.0204, -62.25)
  line L327 (-138.0204, -62.25) -> (-138.0204, -67.75)
  line L328 (-138.0204, -67.75) -> (-143.5204, -67.75)
  line L329 (-143.5204, -67.75) -> (-143.5204, -62.25)
  line L330 (-143.5204, -65) -> (-138.0204, -65) construction
  line L331 (-140.7704, -67.75) -> (-140.7704, -62.25) construction
  line L332 (-108.5204, -62.25) -> (-103.0204, -62.25)
  line L333 (-103.0204, -62.25) -> (-103.0204, -67.75)
  line L334 (-103.0204, -67.75) -> (-108.5204, -67.75)
  line L335 (-108.5204, -67.75) -> (-108.5204, -62.25)
  line L336 (-108.5204, -65) -> (-103.0204, -65) construction
  line L337 (-105.7704, -67.75) -> (-105.7704, -62.25) construction
  line L338 (-353.5204, -97.25) -> (-348.0204, -97.25)
  line L339 (-348.0204, -97.25) -> (-348.0204, -102.75)
  line L340 (-348.0204, -102.75) -> (-353.5204, -102.75)
  line L341 (-353.5204, -102.75) -> (-353.5204, -97.25)
  line L342 (-353.5204, -100) -> (-348.0204, -100) construction
  line L343 (-350.7704, -102.75) -> (-350.7704, -97.25) construction
  line L344 (-318.5204, -97.25) -> (-313.0204, -97.25)
  line L345 (-313.0204, -97.25) -> (-313.0204, -102.75)
  line L346 (-313.0204, -102.75) -> (-318.5204, -102.75)
  line L347 (-318.5204, -102.75) -> (-318.5204, -97.25)
  line L348 (-318.5204, -100) -> (-313.0204, -100) construction
  line L349 (-315.7704, -102.75) -> (-315.7704, -97.25) construction
  line L350 (-283.5204, -97.25) -> (-278.0204, -97.25)
  line L351 (-278.0204, -97.25) -> (-278.0204, -102.75)
  line L352 (-278.0204, -102.75) -> (-283.5204, -102.75)
  line L353 (-283.5204, -102.75) -> (-283.5204, -97.25)
  line L354 (-283.5204, -100) -> (-278.0204, -100) construction
  line L355 (-280.7704, -102.75) -> (-280.7704, -97.25) construction
  line L356 (-248.5204, -97.25) -> (-243.0204, -97.25)
  line L357 (-243.0204, -97.25) -> (-243.0204, -102.75)
  line L358 (-243.0204, -102.75) -> (-248.5204, -102.75)
  line L359 (-248.5204, -102.75) -> (-248.5204, -97.25)
  line L360 (-248.5204, -100) -> (-243.0204, -100) construction
  line L361 (-245.7704, -102.75) -> (-245.7704, -97.25) construction
  line L362 (-213.5204, -97.25) -> (-208.0204, -97.25)
  line L363 (-208.0204, -97.25) -> (-208.0204, -102.75)
  line L364 (-208.0204, -102.75) -> (-213.5204, -102.75)
  line L365 (-213.5204, -102.75) -> (-213.5204, -97.25)
  line L366 (-213.5204, -100) -> (-208.0204, -100) construction
  line L367 (-210.7704, -102.75) -> (-210.7704, -97.25) construction
  line L368 (-178.5204, -97.25) -> (-173.0204, -97.25)
  line L369 (-173.0204, -97.25) -> (-173.0204, -102.75)
  line L370 (-173.0204, -102.75) -> (-178.5204, -102.75)
  line L371 (-178.5204, -102.75) -> (-178.5204, -97.25)
  line L372 (-178.5204, -100) -> (-173.0204, -100) construction
  line L373 (-175.7704, -102.75) -> (-175.7704, -97.25) construction
  line L374 (-143.5204, -97.25) -> (-138.0204, -97.25)
  line L375 (-138.0204, -97.25) -> (-138.0204, -102.75)
  line L376 (-138.0204, -102.75) -> (-143.5204, -102.75)
  line L377 (-143.5204, -102.75) -> (-143.5204, -97.25)
  line L378 (-143.5204, -100) -> (-138.0204, -100) construction
  line L379 (-140.7704, -102.75) -> (-140.7704, -97.25) construction
  line L380 (-108.5204, -97.25) -> (-103.0204, -97.25)
  line L381 (-103.0204, -97.25) -> (-103.0204, -102.75)
  line L382 (-103.0204, -102.75) -> (-108.5204, -102.75)
  line L383 (-108.5204, -102.75) -> (-108.5204, -97.25)
  line L384 (-108.5204, -100) -> (-103.0204, -100) construction
  line L385 (-105.7704, -102.75) -> (-105.7704, -97.25) construction
  point P0 (0, 0)
  point P1 (-350.7704, 145)
  point P2 (-350.7704, 145)
  point P3 (-366.7704, 145)
  point P4 (-350.7704, 161)
  point P5 (-315.7704, 145)
  point P6 (-315.7704, 145)
  point P7 (-280.7704, 145)
  point P8 (-280.7704, 145)
  point P9 (-245.7704, 145)
  point P10 (-245.7704, 145)
  point P11 (-210.7704, 145)
  point P12 (-210.7704, 145)
  point P13 (-175.7704, 145)
  point P14 (-175.7704, 145)
  point P15 (-140.7704, 145)
  point P16 (-140.7704, 145)
  point P17 (-105.7704, 145)
  point P18 (-105.7704, 145)
  point P19 (-350.7704, 110)
  point P20 (-350.7704, 110)
  point P21 (-315.7704, 110)
  point P22 (-315.7704, 110)
  point P23 (-280.7704, 110)
  point P24 (-280.7704, 110)
  point P25 (-245.7704, 110)
  point P26 (-245.7704, 110)
  point P27 (-210.7704, 110)
  point P28 (-210.7704, 110)
  point P29 (-175.7704, 110)
  point P30 (-175.7704, 110)
  point P31 (-140.7704, 110)
  point P32 (-140.7704, 110)
  point P33 (-105.7704, 110)
  point P34 (-105.7704, 110)
  point P35 (-350.7704, 75)
  point P36 (-350.7704, 75)
  point P37 (-315.7704, 75)
  point P38 (-315.7704, 75)
  point P39 (-280.7704, 75)
  point P40 (-280.7704, 75)
  point P41 (-245.7704, 75)
  point P42 (-245.7704, 75)
  point P43 (-210.7704, 75)
  point P44 (-210.7704, 75)
  point P45 (-175.7704, 75)
  point P46 (-175.7704, 75)
  point P47 (-140.7704, 75)
  point P48 (-140.7704, 75)
  point P49 (-105.7704, 75)
  point P50 (-105.7704, 75)
  point P51 (-350.7704, 40)
  point P52 (-350.7704, 40)
  point P53 (-315.7704, 40)
  point P54 (-315.7704, 40)
  point P55 (-280.7704, 40)
  point P56 (-280.7704, 40)
  point P57 (-245.7704, 40)
  point P58 (-245.7704, 40)
  point P59 (-210.7704, 40)
  point P60 (-210.7704, 40)
  point P61 (-175.7704, 40)
  point P62 (-175.7704, 40)
  point P63 (-140.7704, 40)
  point P64 (-140.7704, 40)
  point P65 (-105.7704, 40)
  point P66 (-105.7704, 40)
  point P67 (-350.7704, 5)
  point P68 (-350.7704, 5)
  point P69 (-315.7704, 5)
  point P70 (-315.7704, 5)
  point P71 (-280.7704, 5)
  point P72 (-280.7704, 5)
  point P73 (-245.7704, 5)
  point P74 (-245.7704, 5)
  point P75 (-210.7704, 5)
  point P76 (-210.7704, 5)
  point P77 (-175.7704, 5)
  point P78 (-175.7704, 5)
  point P79 (-140.7704, 5)
  point P80 (-140.7704, 5)
  point P81 (-105.7704, 5)
  point P82 (-105.7704, 5)
  point P83 (-350.7704, -30)
  point P84 (-350.7704, -30)
  point P85 (-315.7704, -30)
  point P86 (-315.7704, -30)
  point P87 (-280.7704, -30)
  point P88 (-280.7704, -30)
  point P89 (-245.7704, -30)
  point P90 (-245.7704, -30)
  point P91 (-210.7704, -30)
  point P92 (-210.7704, -30)
  point P93 (-175.7704, -30)
  point P94 (-175.7704, -30)
  point P95 (-140.7704, -30)
  point P96 (-140.7704, -30)
  point P97 (-105.7704, -30)
  point P98 (-105.7704, -30)
  point P99 (-350.7704, -65)
  point P100 (-350.7704, -65)
  point P101 (-315.7704, -65)
  point P102 (-315.7704, -65)
  point P103 (-280.7704, -65)
  point P104 (-280.7704, -65)
  point P105 (-245.7704, -65)
  point P106 (-245.7704, -65)
  point P107 (-210.7704, -65)
  point P108 (-210.7704, -65)
  point P109 (-175.7704, -65)
  point P110 (-175.7704, -65)
  point P111 (-140.7704, -65)
  point P112 (-140.7704, -65)
  point P113 (-105.7704, -65)
  point P114 (-105.7704, -65)
  point P115 (-350.7704, -100)
  point P116 (-350.7704, -100)
  point P117 (-315.7704, -100)
  point P118 (-315.7704, -100)
  point P119 (-280.7704, -100)
  point P120 (-280.7704, -100)
  point P121 (-245.7704, -100)
  point P122 (-245.7704, -100)
  point P123 (-210.7704, -100)
  point P124 (-210.7704, -100)
  point P125 (-175.7704, -100)
  point P126 (-175.7704, -100)
  point P127 (-140.7704, -100)
  point P128 (-140.7704, -100)
  point P129 (-105.7704, -100)
  point P130 (-105.7704, -100)
  dimension "d21" = 5.5
  dimension "d26" = 35
  dimension "d29" = 35
  constraints: 768 end point, 64 coincident, 7 midpoint, 2 collinear, 2 horizontal, 2 parallel, 2 perpendicular, 1 horizontal alignment, 1 vertical, 1 vertical alignment, 1006 other
  measures "d21" distance of L0.start L0.end
  measures "d26" distance of L0.start L8.start
  measures "d29" distance of L0.start L50.start
extrude "Extrusion5" cut sketch "Sketch5" against normal blind 10
body "Solid1"
